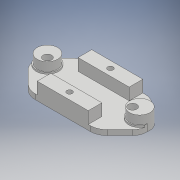
# Autodesk Inventor part: phalanx 2 R F4
Saved by Autodesk Inventor 2017 (Build 210142000, 142)
## iProperties
Created: 2018-07-24
Part Number: phalanx 2 R F4
Material: Generic
Document SubType Name: Modeling
Designer: jakub.tomczynski
Density: 1 g/cm^3
Appearance: Default
Author: jakub.tomczynski
## iProperties of the stored document phalanx 2 R F4_3DPrint.ipt
Created: 2018-09-01
Part Number: phalanx 2 R F4_3DPrint
Material: Generic
Document SubType Name: Modeling
Designer: jakub.tomczynski
Density: 1 g/cm^3
Appearance: Default
Author: jakub.tomczynski
Autodesk Inventor part; units mm, degrees
note: some values were not read from the file. Chosen so that the rebuilt part matches the saved one: arc direction of "baseplate"; arc direction of "Extrusion7".
ref_plane "YZ Plane" through (0, 0, 0) normal (1, 0, 0) x (0, 1, 0)
ref_plane "XZ Plane" through (0, 0, 0) normal (0, 1, 0) x (-1, 0, 0)
ref_plane "XY Plane" through (0, 0, 0) normal (0, 0, 1) x (1, 0, 0)
sketch "axes" plane through (0, 0, 0) normal (0, 0, 1) x (1, 0, 0)
  point P0 (0, 0)
  point P1 (0, 0)
  point P2 (-25, 0)
  dimension "d0" = 25
  constraints: 1 coincident, 1 horizontal alignment
  measures "d0" distance of point (0, 0) point (-25, 0)
sketch "Sketch2" plane through (0, 0, 0) normal (0, 0, 1) x (1, 0, 0)
  circle A0 centre (-25, 0) radius 4
  circle A1 centre (0, 0) radius 4
  line L0 (-22.6569, 8) -> (-2.3431, 8)
  line L1 (-2.3431, -8) -> (-22.6569, -8)
  line L2 (-22.6569, -8) -> (-27.8284, -2.8284)
  line L3 (-22.6569, 8) -> (-27.8284, 2.8284)
  line L4 (-2.3431, 8) -> (2.8284, 2.8284)
  line L5 (-2.3431, -8) -> (2.8284, -2.8284)
  line L6 (-25, 0) -> (0, 0) construction
  dimension "d1" = 8
  dimension "d2" = 8
  dimension "d3" = 16
  dimension "d4" = 45
  dimension "d5" = 45
  constraints: 14 end point, 4 point on circle, 4 tangent, 2 centre point, 2 coincident, 2 horizontal, 2 vertical alignment, 1 parallel, 1 other
  measures "d1" diameter of A0
  measures "d2" diameter of A1
  measures "d3" distance between parallel lines of L1 L0
  measures "d4" angle of L5 L1
  measures "d5" angle of L0 L3
extrude "baseplate" add sketch "Sketch2" along normal blind 1.5
sketch "Sketch3" plane through (0, 0, 1.5) normal (0, 0, 1) x (1, 0, 0)
  arc A0 (-27.8284, 2.8284) -> (-27.8284, -2.8284) centre (-25, 0) ccw projected
  line L0 (-27.8284, -2.8284) -> (-22.6569, -8) projected
  line L1 (-22.6569, -8) -> (-2.3431, -8) projected
  line L2 (-2.3431, -8) -> (2.8284, -2.8284) projected
  arc A1 (2.8284, -2.8284) -> (2.8284, 2.8284) centre (0, 0) ccw projected
  line L3 (2.8284, 2.8284) -> (-2.3431, 8) projected
  line L4 (-2.3431, 8) -> (-22.6569, 8) projected
  line L5 (-22.6569, 8) -> (-27.8284, 2.8284) projected
  line L6 (-20, 8) -> (-5, 8)
  line L7 (-5, 8) -> (-5, 4)
  line L8 (-5, 4) -> (-20, 4)
  line L9 (-20, 4) -> (-20, 8)
  line L10 (-20, -8) -> (-5, -8)
  line L11 (-5, -8) -> (-5, -4)
  line L12 (-5, -4) -> (-20, -4)
  line L13 (-20, -4) -> (-20, -8)
  dimension "d8" = 4
  dimension "d9" = 4
  dimension "d10" = 5
  dimension "d11" = 5
  dimension "d12" = 5
  dimension "d13" = 5
  constraints: 16 end point, 4 parallel, 2 horizontal, 2 perpendicular, 2 point on line
  measures "d8" distance between parallel lines of L10 L12
  measures "d9" distance between parallel lines of L8 L4
  measures "d10" distance from line of L7 point (0, 0)
  measures "d11" distance from line of L9 point (-25, 0)
  measures "d12" distance from line of L13 point (-25, 0)
  measures "d13" distance from line of L11 point (0, 0)
extrude "walls" add sketch "Sketch3" along normal blind 3.5 contours L4 L7 L8 L9 | L13 L12 L11 L1
sketch "Sketch5" plane through (0, 0, 5) normal (0, 0, 1) x (1, 0, 0)
  line L0 (-20, -8) -> (-5, -8) projected
  line L1 (-5, -8) -> (-5, -4) projected
  line L2 (-5, -4) -> (-20, -4) projected
  line L3 (-20, -4) -> (-20, -8) projected
  line L4 (-20, 8) -> (-20, 4) projected
  line L5 (-20, 4) -> (-5, 4) projected
  line L6 (-5, 4) -> (-5, 8) projected
  line L7 (-5, 8) -> (-20, 8) projected
  line L8 (-5, -6) -> (-20, -6) construction
  line L9 (-5, 6) -> (-20, 6) construction
  point P0 (0, 0)
  point P1 (-12.5, -6)
  point P2 (-12.5, 6)
  constraints: 6 midpoint, 4 end point
hole "mounting" at (-12.5, -6, 5) at (-12.5, 6, 5) direction (0, 0, -1) diameter 1.6 depth 4
sketch "Sketch6" plane through (0, 0, 1.5) normal (0, 0, 1) x (1, 0, 0)
  circle A0 centre (1.0607, 1.0607) radius 3
  line L0 (0, 0) -> (1.0607, 1.0607) construction
  line L1 (0, 0) -> (7.1773, 0) construction
  dimension "d30" = 45
  dimension "d31" = 1.5
  dimension "d32" = 6
  constraints: 4 end point, 1 centre point, 1 horizontal
  measures "d30" angle of L1 L0
  measures "d31" distance of L0.end L0.start
  measures "d32" diameter of A0
extrude "pip springy" add sketch "Sketch6" along normal blind 3 and the other way blind 1.5
sketch "Sketch10" plane through (0, 0, 1.5) normal (0, 0, 1) x (1, 0, 0)
  circle A0 centre (1.0607, 1.0607) radius 3 projected
  line L0 (1.6558, 4.001) -> (-2.3431, 8) projected
  arc A1 (2.8284, -2.8284) -> (3.9821, 0.3784) centre (0, 0) ccw projected
  arc A2 (1.36, 4.2968) -> (3.9838, -0.3599) centre (1.0607, 1.0607) ccw
  dimension "d50" = 6.5
  constraints: 3 point on circle, 1 centre point, 1 coincident, 1 point on line
  measures "d50" diameter of A2
extrude "Extrusion7" add sketch "Sketch10" along normal blind 0.5
sketch "Sketch8" plane through (0, 0, 1.5) normal (0, 0, 1) x (1, 0, 0)
  line L0 (-30.1045, 0) -> (-25, 0) construction
  line L1 (-25, 0) -> (-29.2709, 4.2709) construction
  circle A0 centre (-26.0607, 1.0607) radius 3
  point P0 (0, 0)
  dimension "d38" = 45
  dimension "d39" = 6
  dimension "d40" = 1.5
  constraints: 4 end point, 1 centre point, 1 horizontal, 1 point on line
  measures "d38" angle of L1 L0
  measures "d39" diameter of A0
  measures "d40" distance of L0.end A0.centre
extrude "dip springy" add sketch "Sketch8" along normal blind 3 and the other way blind 1.5
sketch "Sketch9" plane through (0, 0, 1.5) normal (0, 0, 1) x (1, 0, 0)
  arc A0 (-28.9821, 0.3784) -> (-26.6558, 4.001) centre (-26.0607, 1.0607) ccw projected
  arc A1 (-28.9838, -0.3599) -> (-26.36, 4.2968) centre (-26.0607, 1.0607) ccw
  line L0 (-22.6569, 8) -> (-26.6558, 4.001) projected
  arc A2 (-28.9821, 0.3784) -> (-27.8284, -2.8284) centre (-25, 0) ccw projected
  point P0 (0, 0)
  dimension "d43" = 6.5
  constraints: 3 point on circle, 1 centre point, 1 coincident, 1 point on line
  measures "d43" diameter of A1
extrude "Extrusion6" add sketch "Sketch9" along normal blind 0.5
sketch "Sketch4" plane through (0, 0, 0) normal (0, 0, -1) x (-1, 0, 0)
  point P0 (25, 0)
  point P1 (0, 0)
hole "joints" at (0, 0, 0) at (-25, 0, 0) direction (0, 0, 1) diameter 2.5 end through all
fillet "Fillet1" radius 5 4 edges at (-2.3431, -8, 0.75) (-22.6569, -8, 0.75) (-22.6569, 8, 0.75) (-2.3431, 8, 0.75)
equation "\"d0\" = PIP_DIP_length"
equation "\"d31\" = PIP_spring_arm"
equation "\"d40\" = DIP_spring_arm"
equation "\"PIP_DIP_length\" = F4_PIP_DIP_length"
equation "\"PIP_spring_arm\" = F4_PIP_spring_arm"
equation "\"DIP_spring_arm\" = F4_DIP_spring_arm"
equation "\"F4_PIP_DIP_length\" = 25"
equation "\"F4_PIP_spring_arm\" = 1.5"
equation "\"F4_DIP_spring_arm\" = 1.5"
body "Solid1"
